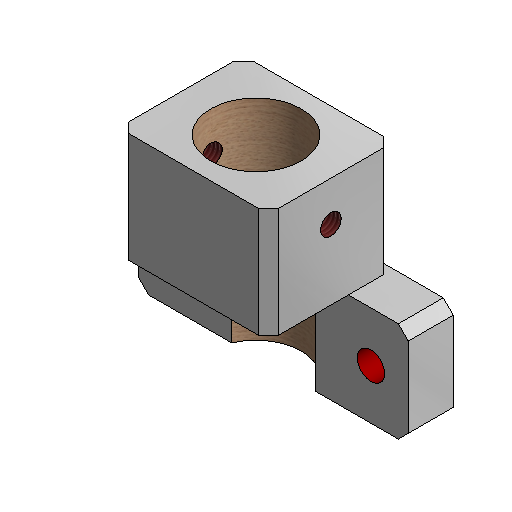
# Autodesk Inventor part: TL20240901-10320CV-026
Saved by Autodesk Inventor 2022.5 (Build 265521000, 521)
## iProperties
Category: FOLLOWER UNIT ASSY
Company: 현대 트랜시스
RuleStatus: InUse
Part Number: TL20240901-10320CV-026
Project: MEa-PJT 2LINE
Checked By: 김형민
Engr Approved By: 김형민
User Status: 2 x6
Material: MC NYLON
Description: 0
Document SubType Name: Modeling
Mfg Approved By: 호상태
Designer: USER106
Stock Number: 026
Density: 0.94 g/cm^3
Appearance: MC NYLON(백색)
Detail Description: Processed products
Title: SENSOR HOLDER
Subject: MEa차종 시트조립2라인
Author: USER106
Revision Number: A
Autodesk Inventor part; units mm, degrees
ref_plane "YZ Plane" through (0, 0, 0) normal (1, 0, 0) x (0, 1, 0)
ref_plane "XZ Plane" through (0, 0, 0) normal (0, 1, 0) x (-1, 0, 0)
ref_plane "XY Plane" through (0, 0, 0) normal (0, 0, 1) x (1, 0, 0)
sketch "Sketch7" plane through (0, 0, 0) normal (0, 0, 1) x (1, 0, 0)
  line L0 (15, -12.5) -> (-15, -12.5)
  line L1 (-15, -12.5) -> (-15, 12.5)
  line L2 (-15, 12.5) -> (15, 12.5)
  line L3 (15, 12.5) -> (15, -12.5)
  line L4 (15, -12.5) -> (-15, 12.5) construction
  line L5 (-15, -12.5) -> (15, 12.5) construction
  point P0 (0, 0)
  dimension "d26" = 30
  dimension "d27" = 25
  constraints: 12 end point, 2 midpoint, 2 parallel, 1 horizontal, 1 perpendicular
  measures "d26" distance of L1.end L2.end
  measures "d27" distance of L0.end L1.end
extrude "Extrusion4" add sketch "Sketch7" along normal blind 22
sketch "Sketch8" plane through (0, 0, 0) normal (0, 0, -1) x (-1, 0, 0)
  line L0 (-27, 12.5) -> (27, 12.5)
  line L1 (27, 12.5) -> (27, 3.5)
  line L2 (27, 3.5) -> (-27, 3.5)
  line L3 (-27, 3.5) -> (-27, 12.5)
  line L4 (-15, -12.5) -> (-15, 12.5) projected
  line L5 (15, 12.5) -> (15, -12.5) projected
  line L6 (-15, 12.5) -> (15, 12.5) projected
  point P0 (0, 0)
  dimension "d30" = 12
  dimension "d31" = 12
  dimension "d32" = 9
  constraints: 8 end point, 2 parallel, 1 horizontal, 1 perpendicular, 1 point on line
  measures "d30" distance between parallel lines of L3 L4
  measures "d31" distance between parallel lines of L1 L5
  measures "d32" distance between parallel lines of L0 L2
extrude "Extrusion5" add sketch "Sketch8" along normal blind 20
sketch "Sketch9" plane through (0, 0, 22) normal (0, 0, 1) x (1, 0, 0)
  line L0 (15, 12.5) -> (-15, 12.5) projected
  line L1 (15, -12.5) -> (15, 12.5) projected
  point P0 (0, 0)
  point P1 (0, 0)
  point P2 (0, 12.5)
  point P3 (15, 0)
  constraints: 2 midpoint, 1 horizontal alignment, 1 vertical alignment
hole "Hole3" at (0, 0, 22) direction (0, 0, -1) diameter 18.1 end through all
sketch "Sketch10" plane through (15, 3.5, 0) normal (0, -1, 0) x (1, 0, 0)
  line L0 (12, 0) -> (0, 0) projected
  line L1 (12, -20) -> (-6.6542, -20) projected
  line L2 (12, 0) -> (12, -20) projected
  line L3 (-42, 0) -> (-42, -20) projected
  point P0 (-15, 0)
  point P1 (4.5, -10)
  point P2 (-34.5, -10)
  dimension "d42" = 20
  dimension "d43" = 10
  dimension "d44" = 7.5
  dimension "d45" = 7.5
  constraints: 1 horizontal alignment
  measures "d42" distance between parallel lines of L0 L1
  measures "d43" distance from line of point (4.5, -10) L1
  measures "d44" distance from line of point (4.5, -10) L2
  measures "d45" distance from line of point (-34.5, -10) L3
hole "Hole4" at (19.5, 3.5, -10) at (-19.5, 3.5, -10) direction (0, 1, 0) diameter 5.5 end through all clearance for "Socket Head Cap Screw" size "M5" standard "TS Profile"
chamfer "Chamfer1" distance 2 angle 45 8 edges at (15, 12.5, 11) (15, -12.5, 11) (-15, -12.5, 11) (-15, 12.5, 11) (27, 8, 0) (27, 8, -20) (-27, 8, -20) (-27, 8, 0)
sketch "Sketch11" plane through (15, -10.5, 0) normal (1, 0, 0) x (0, 0, -1)
  line L0 (-22, 0) -> (-22, 21) projected
  point P0 (0, 10.5)
  point P1 (-14, 10.5)
  dimension "d63" = 8
  constraints: 1 horizontal alignment
  measures "d63" distance from line of point (-14, 10.5) L0
hole "Hole5" at (15, 0, 14) direction (-1, 0, 0) diameter 4.134 end through all thread size "M5x0.8" class "6H" standard "TS profile"
equation "\"d31\" = d30"
equation "\"d43\" = 0.5 * d42"
equation "\"d45\" = d44"
body "Solid3"
